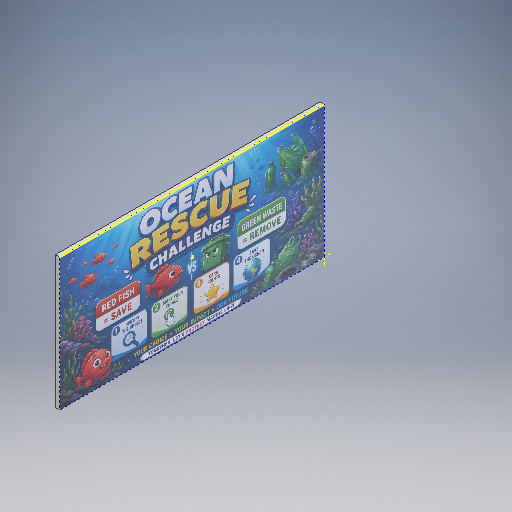
# Autodesk Inventor part: game board
Saved by Autodesk Inventor 2025.3 (Build 293356000, 356)
## iProperties
Created: 2026-06-11
Part Number: game board
Material: Generic
Document SubType Name: Modeling
Designer: user
Density: 1 g/cm^3
Appearance: Default
Author: user
Autodesk Inventor part; units mm, degrees
ref_plane "YZ Plane" through (0, 0, 0) normal (1, 0, 0) x (0, 1, 0)
ref_plane "XZ Plane" through (0, 0, 0) normal (0, 1, 0) x (-1, 0, 0)
ref_plane "XY Plane" through (0, 0, 0) normal (0, 0, 1) x (1, 0, 0)
sketch "Sketch1" plane through (0, 0, 0) normal (1, 0, 0) x (0, 1, 0)
  line L0 (-150, 300) -> (150, 300)
  line L1 (150, 300) -> (150, -300)
  line L2 (150, -300) -> (-150, -300)
  line L3 (-150, -300) -> (-150, 300)
  line L4 (-150, 300) -> (150, -300) construction
  line L5 (150, 300) -> (-150, -300) construction
  point P0 (0, 0)
  dimension "d0" = 300
  dimension "d1" = 600
  constraints: 12 end point, 2 midpoint, 2 parallel, 1 horizontal, 1 perpendicular
  measures "d0" distance of L1.end L2.end
  measures "d1" distance of L0.end L1.end
extrude "Extrusion1" add sketch "Sketch1" along normal blind 10
sketch "Sketch2" plane through (10, 0, 0) normal (1, 0, 0) x (0, 0, -1)
  line L0 (300, 150) -> (-300, 150) projected
  line L1 (-300, 150) -> (300, 150) construction
  line L2 (300, 150) -> (300, -150) construction
  line L3 (300, -150) -> (-300, -150) construction
  line L4 (-300, -150) -> (-300, 150) construction
  point P0 (0, 0)
  constraints: 1 coincident, 2 other
body "Solid1"
